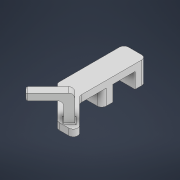
# Autodesk Inventor part: NozzleCleaner
Saved by Autodesk Inventor 2022 (Build 260153000, 153)
## iProperties
Created: 2024-01-20
Part Number: NozzleCleaner
Material: Všeobecné
Document SubType Name: Modeling
Designer: tada
Density: 1 g/cm^3
Appearance: Výchozí
Author: tada
Autodesk Inventor part; units mm, degrees
ref_plane "YZ Plane" through (0, 0, 0) normal (1, 0, 0) x (0, 1, 0)
ref_plane "XZ Plane" through (0, 0, 0) normal (0, 1, 0) x (-1, 0, 0)
ref_plane "XY Plane" through (0, 0, 0) normal (0, 0, 1) x (1, 0, 0)
sketch "Náčrt1" plane through (0, 0, 0) normal (0, 1, 0) x (-1, 0, 0)
  line L0 (0, 0) -> (-10, 0)
  line L1 (-10, 0) -> (-10, -5)
  line L2 (-10, -5) -> (0, -5)
  line L3 (0, -5) -> (0, 0)
  line L4 (0, -15) -> (-10, -15)
  line L5 (-10, -15) -> (-10, -20)
  line L6 (-10, -20) -> (0, -20)
  line L7 (0, -20) -> (0, -15)
  dimension "d0" = 10
  dimension "d1" = 5
  dimension "d2" = 5
  dimension "d3" = 10
  constraints: 16 end point, 4 parallel, 2 horizontal, 2 perpendicular, 2 point on line
  measures "d0" distance between parallel lines of L4 L2
  measures "d1" distance of L2.end L0.start
  measures "d2" distance of L6.end L4.start
  measures "d3" distance of L5.end L6.end
extrude "Vysunutí1" add sketch "Náčrt1" along normal blind 7
sketch "Náčrt2" plane through (0, 7, 0) normal (0, 1, 0) x (1, 0, 0)
  line L0 (0, 0) -> (10, 0)
  line L1 (10, 0) -> (10, 20)
  line L2 (10, 20) -> (0, 20)
  line L3 (0, 20) -> (0, 0)
  line L4 (10, 0) -> (10, 5) projected
  line L5 (10, 0) -> (0, 0)
  line L6 (0, 0) -> (0, -10)
  line L7 (0, -10) -> (10, -10)
  line L8 (10, -10) -> (10, 0)
  line L9 (10, -10) -> (25, -25)
  line L10 (0, -10) -> (15, -25)
  line L11 (25, -25) -> (15, -25)
  dimension "d6" = 10
  dimension "d7" = 10
  dimension "d8" = 135
  dimension "d9" = 15
  dimension "d10" = 15
  constraints: 22 end point, 5 parallel, 2 horizontal, 2 perpendicular
  measures "d6" distance of L5.end L6.end
  measures "d7" distance between parallel lines of L8 L6
  measures "d8" angle of L9 L8
  measures "d9" horizontal distance of L7.end L9.end
  measures "d10" horizontal distance of L6.end L10.end
extrude "Vysunutí2" add sketch "Náčrt2" along normal blind 3
sketch "Náčrt3" plane through (0, 10, 0) normal (0, 1, 0) x (1, 0, 0)
  line L0 (15, -25) -> (25, -25)
  line L1 (17.328427, -24.5) -> (14.828427, -22)
  line L2 (14.828427, -22) -> (17.328427, -19.5)
  line L3 (17.328427, -19.5) -> (19.828427, -22)
  line L4 (19.828427, -22) -> (17.328427, -24.5)
  line L5 (0, -10) -> (15, -25)
  point P0 (0, 0)
  dimension "d22" = 2.5
  dimension "d23" = 2.5
  dimension "d24" = 0.5
  dimension "d25" = 2
  constraints: 8 end point, 3 perpendicular, 1 parallel
  measures "d22" horizontal distance of L1.start L1.end
  measures "d23" horizontal distance of L1.end L2.end
  measures "d24" distance from line of L1.start L0
  measures "d25" distance from line of L5 L1.end
extrude "Vysunutí5" add sketch "Náčrt3" along normal blind 12
sketch "Náčrt5" plane through (17.328427, 10, 24.5) normal (-0.7071068, 0, 0.7071068) x (0.7071068, 0, 0.7071068)
  line L0 (0, 12) -> (-3.535534, 12)
  line L1 (0, 0) -> (0, 12)
  line L2 (-3.535534, 12) -> (0, 12)
  line L3 (0, 12) -> (0, 9)
  line L4 (0, 9) -> (-3.535534, 9)
  line L5 (-3.535534, 9) -> (-3.535534, 12)
  point P0 (-29.577164, -10)
  dimension "d28" = 3
  constraints: 8 end point, 2 parallel, 1 horizontal, 1 perpendicular, 1 point on line
  measures "d28" distance between parallel lines of L4 L0
extrude "Vysunutí6" add sketch "Náčrt5" along normal blind 12
fillet "Zaoblení1" radius 2 8 edges at (25, 8.5, 25) (15, 8.5, 25) (10, 8.5, 10) (0, 8.5, 10) (10, 5, -20) (0, 5, -20) (0, 3.5, 0) (10, 3.5, 0)
fillet "Zaoblení2" radius 2 1 edges at (16.0784, 19, 23.25)
fillet "Zaoblení3" radius 0.5 4 edges at (16.0784, 10, 20.75) (16.0784, 10, 23.25) (18.5784, 10, 20.75) (18.5784, 10, 23.25)
fillet "Zaoblení4" radius 2 1 edges at (18.5784, 22, 20.75)
fillet "Zaoblení5" radius 0.5 4 edges at (7.5931, 22, 31.7353) (7.5931, 19, 31.7353) (8.8431, 20.5, 32.9853) (6.3431, 20.5, 30.4853)
equation "\"d10\" = d9"
